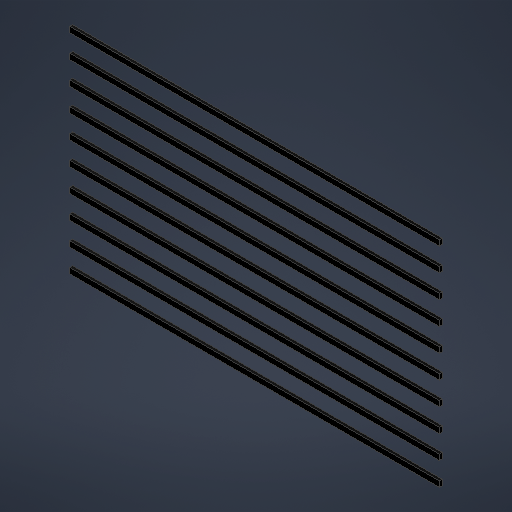
# Autodesk Inventor part: rampbands
Saved by Autodesk Inventor 2026.1 (Build 301233000, 233)
## iProperties
Created: 2025-11-04
Part Number: rampbands
Material: Generic
Document SubType Name: Modeling
Designer: roejo
Density: 1 g/cm^3
Appearance: Default
Author: roejo
Autodesk Inventor part; units mm, degrees
ref_plane "YZ Plane" through (0, 0, 0) normal (1, 0, 0) x (0, 1, 0)
ref_plane "XZ Plane" through (0, 0, 0) normal (0, 1, 0) x (-1, 0, 0)
ref_plane "XY Plane" through (0, 0, 0) normal (0, 0, 1) x (1, 0, 0)
sketch "Sketch1" plane through (0, 0, 0) normal (0, 0, 1) x (1, 0, 0)
  line L0 (-6.1499, 1.3208) -> (196.1611, 1.3208)
  line L1 (196.1611, 1.3208) -> (196.1611, 4.3688)
  line L2 (196.1611, 4.3688) -> (-6.1499, 4.3688)
  line L3 (-6.1499, 4.3688) -> (-6.1499, 1.3208)
  line L4 (-6.1499, 14.0208) -> (196.1611, 14.0208)
  line L5 (196.1611, 14.0208) -> (196.1611, 17.0688)
  line L6 (196.1611, 17.0688) -> (-6.1499, 17.0688)
  line L7 (-6.1499, 17.0688) -> (-6.1499, 14.0208)
  line L8 (196.1611, 29.7688) -> (-6.1499, 29.7688)
  line L9 (-6.1499, 26.7208) -> (196.1611, 26.7208)
  line L10 (-6.1499, 29.7688) -> (-6.1499, 26.7208)
  line L11 (196.1611, 26.7208) -> (196.1611, 29.7688)
  line L12 (196.1611, 42.4688) -> (-6.1499, 42.4688)
  line L13 (-6.1499, 39.4208) -> (196.1611, 39.4208)
  line L14 (-6.1499, 42.4688) -> (-6.1499, 39.4208)
  line L15 (196.1611, 39.4208) -> (196.1611, 42.4688)
  line L16 (196.1611, 55.1688) -> (-6.1499, 55.1688)
  line L17 (-6.1499, 52.1208) -> (196.1611, 52.1208)
  line L18 (-6.1499, 55.1688) -> (-6.1499, 52.1208)
  line L19 (196.1611, 52.1208) -> (196.1611, 55.1688)
  line L20 (196.1611, 67.8688) -> (-6.1499, 67.8688)
  line L21 (-6.1499, 64.8208) -> (196.1611, 64.8208)
  line L22 (-6.1499, 67.8688) -> (-6.1499, 64.8208)
  line L23 (196.1611, 64.8208) -> (196.1611, 67.8688)
  line L24 (196.1611, 80.5688) -> (-6.1499, 80.5688)
  line L25 (-6.1499, 77.5208) -> (196.1611, 77.5208)
  line L26 (-6.1499, 80.5688) -> (-6.1499, 77.5208)
  line L27 (196.1611, 77.5208) -> (196.1611, 80.5688)
  line L28 (196.1611, 93.2688) -> (-6.1499, 93.2688)
  line L29 (-6.1499, 90.2208) -> (196.1611, 90.2208)
  line L30 (-6.1499, 93.2688) -> (-6.1499, 90.2208)
  line L31 (196.1611, 90.2208) -> (196.1611, 93.2688)
  line L32 (196.1611, 105.9688) -> (-6.1499, 105.9688)
  line L33 (-6.1499, 102.9208) -> (196.1611, 102.9208)
  line L34 (-6.1499, 105.9688) -> (-6.1499, 102.9208)
  line L35 (196.1611, 102.9208) -> (196.1611, 105.9688)
  line L36 (196.1611, 118.6688) -> (-6.1499, 118.6688)
  line L37 (-6.1499, 115.6208) -> (196.1611, 115.6208)
  line L38 (-6.1499, 118.6688) -> (-6.1499, 115.6208)
  line L39 (196.1611, 115.6208) -> (196.1611, 118.6688)
  point P0 (0, 0)
  dimension "d0" = 202.311
  dimension "d1" = 3.048
  dimension "d2" = 12.7
  dimension "d3" = 202.311
  dimension "d4" = 3.048
  dimension "d7" = 12.7
  constraints: 80 end point, 4 parallel, 2 horizontal, 2 perpendicular, 1 collinear, 1 vertical, 63 other
  measures "d0" distance of L2.end L1.end
  measures "d1" distance of L1.end L0.end
  measures "d2" distance of L0.start L4.start
  measures "d3" distance of L6.end L5.end
  measures "d4" distance of L5.end L4.end
  measures "d7" distance of L5.end L8.start
extrude "Extrusion1" add sketch "Sketch1" along normal blind 1.5875
body "Solid1"
